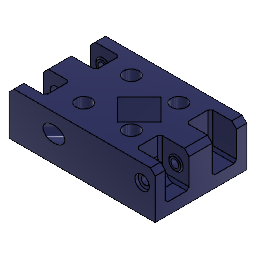
1-Xaxis_Mount_Right v2 v1 (Autodesk Fusion 360 design; units mm, degrees)
Autodesk Fusion 360 part; units mm, degrees
mesh "Mesh1" [no effect]
sketch "Mesh Selection Sketch XY 16mm" plane through (0, 0, 16) normal (0, 0, 1) x (1, 0, 0)
sketch "Sketch XY" plane through (0, 0, 0) normal (0, 0, 1) x (1, 0, 0)
  circle A0 centre (-9, 10.4) radius 3.25
  line L0 (-30.75, 19.3) -> (30.75, 19.3)
  line L1 (30.75, 19.3) -> (30.75, -19.3)
  line L2 (30.75, -19.3) -> (-30.75, -19.3)
  line L3 (-30.75, -19.3) -> (-30.75, 19.3)
  line L4 (-30.75, 14.9) -> (-18.45, 14.9)
  line L5 (-18.45, 14.9) -> (-18.45, 4.9)
  line L6 (-18.45, 4.9) -> (-30.75, 4.9)
  line L7 (-30.75, 0) -> (30.75, 0) construction
  circle A1 centre (-9, 10.4) radius 1.6
  circle A2 centre (-9, 10.4) radius 3.25
  circle A3 centre (-9, 10.4) radius 1.6
  circle A4 centre (11, 10.4) radius 3.25
  circle A5 centre (11, 10.4) radius 1.6
  circle A6 centre (-9, -9.6) radius 3.25
  circle A7 centre (-9, -9.6) radius 1.6
  circle A8 centre (11, -9.6) radius 3.25
  circle A9 centre (11, -9.6) radius 1.6
  line L8 (30.75, -15.05) -> (18.45, -15.05)
  line L9 (18.45, -15.05) -> (18.45, -5.05)
  line L10 (18.45, -5.05) -> (30.75, -5.05)
  line L11 (30.75, 14.9) -> (19.75, 14.9)
  line L12 (19.75, 14.9) -> (19.75, 4.65)
  line L13 (19.75, 4.65) -> (30.75, 4.65)
  line L14 (-30.75, -4.8) -> (-19.75, -4.8)
  line L15 (-19.75, -4.8) -> (-19.75, -15.05)
  line L16 (-19.75, -15.05) -> (-30.75, -15.05)
  line L17 (5.1492, 8.679) -> (14.2708, -0.4427)
  line L18 (14.2708, -0.4427) -> (5.1492, -9.5644)
  line L19 (5.1492, -9.5644) -> (-3.9725, -0.4427)
  line L20 (-3.9725, -0.4427) -> (5.1492, 8.679)
  dimension "d1" = 6.5
  dimension "d2" = 61.5
  dimension "d3" = 38.6
  dimension "d4" = 10
  dimension "d5" = 12.3
  dimension "d6" = 4.4
  dimension "d7" = 9
  dimension "d8" = 10.4
  dimension "d9" = 3.2
  dimension "d10" = 6.5
  dimension "d11" = 3.2
  dimension "d14" = 20
  dimension "d15" = -20
  dimension "d17" = 4.4
  dimension "d18" = 4.25
  dimension "d19" = 4.25
  dimension "d20" = 11
  dimension "d21" = 10.25
  dimension "d22" = 30.75
  dimension "d23" = 45
  dimension "d26" = 0.4427
  dimension "d27" = 12.9
  dimension "d28" = 3.9725
  dimension "d29" = 12.9
  constraint horizontal L0
  constraint vertical L1
  constraint horizontal L2
  constraint vertical L3
  constraint horizontal L4
  constraint vertical L5
  constraint horizontal L6
  constraint coincident L3 L4.start
  constraint midpoint L3 L7.start
  constraint midpoint L1 L7.end
  constraint coincident origin L7
  constraint concentric A0 A1
  constraint concentric A2 A3
  constraint coincident L1 L8.start
  constraint perpendicular L1 L8
  constraint perpendicular L8 L9
  constraint coincident L1 L10.end
  constraint perpendicular L1 L10
  constraint coincident L1 L11.start
  constraint perpendicular L1 L11
  constraint perpendicular L11 L12
  constraint coincident L1 L13.end
  constraint perpendicular L1 L13
  constraint coincident L3 L14.start
  constraint perpendicular L3 L14
  constraint perpendicular L14 L15
  constraint coincident L3 L16.end
  constraint perpendicular L3 L16
  constraint perpendicular L17 L18
  constraint parallel L17 L19
  constraint parallel L18 L20
  constraint equal L5 L9
  constraint equal L6 L8
  constraint equal L4 L10
  constraint equal L12 L15
  constraint equal L11 L14
  measures "d1" diameter of A0
  measures "d2" distance of L0.start L0.end
  measures "d3" distance of L0.start L2.end
  measures "d4" distance of L4.start L6.end
  measures "d5" distance of L4.start L4.end
  measures "d6" distance of L0 L4
  measures "d7" horizontal distance of origin A0.centre
  measures "d8" vertical distance of origin A0.centre
  measures "d9" diameter of A1
  measures "d10" diameter of A2
  measures "d11" diameter of A3
  measures "d17" distance of L0 L11
  measures "d18" distance of L2 L16
  measures "d19" distance of L2 L8
  measures "d20" distance of L15.end L16.end
  measures "d21" distance of L14.end L15.end
  measures "d22" distance of origin L1
  measures "d23" angle of L7 L20
  measures "d26" distance of L7 L19.end
  measures "d27" distance of L17.start L19.end
  measures "d28" horizontal distance of origin L19.end
  measures "d29" distance of L18.end L19.end
extrude "Extrude1" add sketch "Sketch XY" along normal blind 19 contours A0 A2 | L0 L1 L2 L3 L4 L5 L6 L8 L9 L10 L11 L12 L13 L14 L15 L16 | L3 L4 L5 L6 | L1 L11 L12 L13 | L3 L14 L15 L16 | L1 L8 L9 L10 | A4 | A6 | A8 | L17 L18 L19 L20
extrude "Extrude2" cut sketch "Sketch XY" against normal blind 14 from surface at 19 contours L3 L4 L5 L6 | L1 L11 L12 L13 | L3 L14 L15 L16 | L1 L8 L9 L10
extrude "Extrude3" cut sketch "Sketch XY" against normal blind 12 from surface at 19 contours L17 L18 L19 L20
extrude "Extrude4" cut sketch "Sketch XY" against normal blind 5 from surface at 19 contours A0 A2 | A4 | A6 | A8
sketch "Mesh Selection Sketch XZ" plane through (0, 0, 0) normal (0, 1, 0) x (-1, 0, 0)
sketch "Sketch Side holes" plane through (0, 0, 0) normal (0, 1, 0) x (1, 0, 0)
  circle A0 centre (-25.4, -11.9) radius 2.5
  circle A1 centre (25.25, -11.9) radius 2.5
  circle A2 centre (-25.4, -11.9) radius 1.6
  circle A3 centre (-25.4, -11.9) radius 3
  circle A4 centre (25.25, -11.9) radius 1.6
  circle A5 centre (25.25, -11.9) radius 3
  dimension "d41" = 5
  dimension "d43" = 25.4
  dimension "d45" = 25.25
  dimension "d46" = 3.2
  dimension "d47" = 6
  dimension "d48" = 11.9
  constraint equal A0 A1
  constraint horizontal A0.centre A1.centre
  constraint concentric A0 A2
  constraint concentric A0 A3
  constraint concentric A1 A4
  constraint concentric A4 A5
  constraint equal A2 A4
  constraint equal A3 A5
  measures "d41" diameter of A0
  measures "d43" horizontal distance of A0.centre origin
  measures "d45" horizontal distance of origin A1.centre
  measures "d46" diameter of A2
  measures "d47" diameter of A3
  measures "d48" vertical distance of origin A0.centre
extrude "Extrude5" cut sketch "Sketch Side holes" along normal up to surface (19.3 mm away) and the other way up to surface (4.8 mm away) contours A2
extrude "Extrude6" cut sketch "Sketch Side holes" against normal up to surface (4.8 mm away) contours A0
extrude "Extrude7" cut sketch "Sketch Side holes" against normal blind 1.5 from surface at 19.3 contours A0 | A3
extrude "Extrude8" add sketch "Sketch Side holes" along normal blind 0.5 from surface at 4.9 contours A0
extrude "Extrude9" add sketch "Sketch Side holes" against normal blind 0.5 from surface at 14.9 contours A0
extrude "Extrude10" cut sketch "Sketch Side holes" along normal up to surface (4.65 mm away) and the other way up to surface (19.3 mm away) contours A4
extrude "Extrude11" cut sketch "Sketch Side holes" along normal up to surface (4.65 mm away) contours A1
extrude "Extrude12" cut sketch "Sketch Side holes" along normal blind 1.3 from surface at -19.3 contours A1 | A5
extrude "Extrude13" add sketch "Sketch Side holes" against normal blind 0.5 from surface at -5.05 contours A1
extrude "Extrude14" add sketch "Sketch Side holes" along normal blind 0.5 from surface at -15.05 contours A1
sketch "Sketch5" plane through (-1.7993, -4.0275, 11.4257) normal (0.707107, 0.707107, 0) x (-0.707107, 0.707107, 0)
ref_plane "WorkPlane1" through (0, 0, 12.125) normal (0.707107, 0.707107, 0) x (0, 0, 1)
sketch "Sketch6" plane through (0, 0, 12.125) normal (0.707107, 0.707107, 0) x (0, 0, 1)
  circle A0 centre (-1.125, 5.25) radius 1.5
  circle A1 centre (-1.125, 5.25) radius 3.25
  point P0 (-12.125, 0)
  dimension "d81" = 3
  dimension "d82" = 11
  dimension "d83" = 5.25
  dimension "d84" = 6.5
  constraint concentric A0 A1
  measures "d81" diameter of A0
  measures "d82" horizontal distance of A0.centre P0
  measures "d83" vertical distance of A0.centre P0
  measures "d84" diameter of A1
extrude "Extrude15" cut sketch "Sketch6" along normal up to surface contours A0 end surface through (30.75, -19.3, 0) normal (0, -1, 0) offset 0
extrude "Extrude16" cut sketch "Sketch6" along normal up to surface from surface at -11 end surface through (30.75, -19.3, 0) normal (0, -1, 0) offset 0
chamfer "Chamfer1" distance 2 angle 45 6 edges at (30.75, -17.175, 19) (30.75, -0.2, 19) (30.75, 17.1, 19) (-30.75, 17.1, 19) (-30.75, 0.05, 19) (-30.75, -17.175, 19)
chamfer "Chamfer2" distance 1 angle 45 18 edges at (25.25, 4.65, 5) (19.75, 9.775, 5) (25.25, 14.9, 5) (24.6, -15.05, 5) (24.6, -5.05, 5) (18.45, -15.05, 12) (18.45, -5.05, 12) (19.75, 4.65, 12) (19.75, 14.9, 12) (-18.45, 4.9, 12) (-18.45, 14.9, 12) (-24.6, 4.9, 5) (-24.6, 14.9, 5) (-19.75, -15.05, 12) (-19.75, -4.8, 12) (-19.75, -9.925, 5) (-25.25, -15.05, 5) (-25.25, -4.8, 5)
fillet "Fillet2" radius 6.5 2 edges at (-18.45, 9.9, 5) (18.45, -10.05, 5)
chamfer "Chamfer3" distance 0.5 angle 45 4 edges at (22.9192, -5.05, 12.804) (22.9192, -15.05, 10.996) (-27.7308, 4.9, 10.996) (-27.7308, 14.9, 12.804)
equation "d17 = d6"
equation "d19 = d18"
equation "d22 = d2 / 2"
